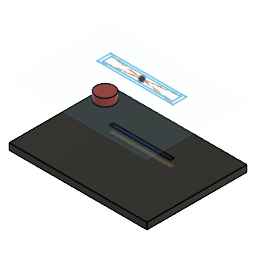
Top (Autodesk Fusion 360 design; units mm, degrees)
part number: 2026-05-12-00-53-40-526
Autodesk Fusion 360 part; units mm, degrees
note: some values were not read from the file. Set by a fixed rule: which sketch regions a step uses.
sketch "Sketch1" plane through (0, 0, 0) normal (0, 0, 1) x (1, 0, 0)
  line L0 (-63.249, 34) -> (63.7766, 34)
  line L1 (63.7766, 34) -> (63.7766, -58)
  line L2 (63.7766, -58) -> (-63.249, -58)
  line L3 (-63.249, -58) -> (-63.249, 34)
  line L4 (25.177, 2.3381) -> (-31.177, 2.3381)
  line L5 (-31.177, 2.3381) -> (-31.177, 5.636)
  line L6 (-31.177, 5.636) -> (25.177, 5.636)
  line L7 (25.177, 5.636) -> (25.177, 2.3381)
  line L8 (25.177, 2.3381) -> (-31.177, 5.636) construction
  line L9 (-31.177, 2.3381) -> (25.177, 5.636) construction
  line L10 (0.2638, 34) -> (0.2638, -58)
  circle A0 centre (-53.4288, 20.5672) radius 8.3963
  line L11 (-57.7913, -53.2882) -> (58.1506, -53.2882)
  line L12 (58.1506, -53.2882) -> (58.1506, 29.1652)
  line L13 (58.1506, 29.1652) -> (-57.7913, 29.1652)
  line L14 (-57.7913, 29.1652) -> (-57.7913, -53.2882)
  point P0 (-3, 3.987)
  point P1 (1.8186, -10.5131)
  dimension "d7" = 92
  constraint horizontal L0
  constraint vertical L1
  constraint horizontal L2
  constraint vertical L3
  constraint horizontal L4
  constraint perpendicular L4 L5
  constraint parallel L4 L6
  constraint parallel L5 L7
  constraint coincident L8 P0
  constraint coincident L9 P0
  constraint midpoint L0 L10.start
  constraint midpoint L2 L10.end
  constraint horizontal L11
  constraint vertical L12
  constraint horizontal L13
  constraint vertical L14
  measures "d7" distance of L0.end L1.end
extrude "Extrude1" add sketch "Sketch1" along normal blind 6 contours L0 L2 L3 L10 A0 L11 L13 L14 | L0 L1 L2 L10 L11 L12 L13 | L4 L6 L7 L10 L11 L12 L13 | L4 L5 L6 L10 A0 L11 L13 L14 | A0 L14 | A0 L14 makes body 1
extrude "Extrude2" add sketch "Sketch1" along normal blind 13 contours A0 L14 | A0 L14 bodies 1
move_body "Move1" bodies 1 to x (1, 0, 0) y (0, 1, 0) z (0, 0, 1) at (0, 0, 130)
sketch "Sketch2" plane through (0, 0, 136) normal (0, 0, 1) x (-1, 0, 0)
  circle A0 centre (53.4288, -20.5672) radius 8.3963
  line L0 (31.177, -5.636) -> (-25.177, -5.636)
  line L1 (-25.177, -5.636) -> (-25.177, -2.3381)
  line L2 (-25.177, -2.3381) -> (31.177, -2.3381)
  line L3 (31.177, -2.3381) -> (31.177, -5.636)
  line L4 (63.249, 58) -> (-63.7766, 58)
  line L5 (-63.7766, 58) -> (-63.7766, -34)
  line L6 (-63.7766, -34) -> (63.249, -34)
  line L7 (63.249, -34) -> (63.249, 58)
  line L8 (-29, 0) -> (35, 0)
  line L9 (35, 0) -> (35, -8)
  line L10 (35, -8) -> (-29, -8)
  line L11 (-29, -8) -> (-29, 0)
  line L12 (-29, 0) -> (35, -8) construction
  line L13 (35, 0) -> (-29, -8) construction
  line L14 (-31.9009, 2.1844) -> (37.9009, 2.1844)
  line L15 (37.9009, 2.1844) -> (37.9009, -10.1844)
  line L16 (37.9009, -10.1844) -> (-31.9009, -10.1844)
  line L17 (-31.9009, -10.1844) -> (-31.9009, 2.1844)
  line L18 (-31.9009, 2.1844) -> (37.9009, -10.1844) construction
  line L19 (37.9009, 2.1844) -> (-31.9009, -10.1844) construction
  point P0 (3, -4)
  point P1 (3, -4)
  constraint horizontal L8
  constraint perpendicular L8 L9
  constraint parallel L8 L10
  constraint parallel L9 L11
  constraint coincident L12 P1
  constraint coincident L13 P1
  constraint horizontal L14
  constraint perpendicular L14 L15
  constraint parallel L14 L16
  constraint parallel L15 L17
  constraint coincident L18 P1
  constraint coincident L19 P1
  constraint coincident P1 P0
extrude "Extrude6" add sketch "Sketch1" along normal blind 2.5 separate body contours L4 L6 L7 L10 L11 L12 L13 | L4 L5 L6 L10 A0 L11 L13 L14 | A0 L14 picked at (-47.8272, 18.9839) makes body 2
move_body "Move3" bodies 2 to x (1, 0, 0) y (0, 1, 0) z (0, 0, 1) at (0, 0, 127)
move_body "Move4" bodies 1 2 to x (1, 0, 0) y (0, 1, 0) z (0, 0, 1) at (0, 0, -50)
